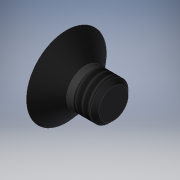
# Autodesk Inventor part: FBb4-5
Saved by Autodesk Inventor 2019 (Build 230136000, 136)
## iProperties
Created: 2024-03-12
Part Number: FBb4-5
Material: Generic
Catalog Web Link: www.cadenas.de
Description: FBb-Cross Recessed Countersunk Head Screw
Vendor: MISUMI
Document SubType Name: Modeling
Designer: psAdmin
Manufacturer: MISUMI
Mass: 0.0947838 g
Surface Area: 1.75917 cm^2
Volume: 0.0947838 cm^3
Density: 1 g/cm^3
Appearance: PSOLRGB-175-175-175
Category: PARTsolutions
Company: MISUMI
Title: FBb4-5
Author: Cadenas PARTsolutions
Comments: Cross Recessed Countersunk Head Screw
PSOL_IDENT_0: {$CADENAS_DATA/23d-libs/misumi/metric/28_keys_magnets/fb_b.prj},152 {VTYP=3D},{NB=FBb4-5},{LINA=FBb4
PSOL_IDENT_1: -5},{NN=FBb},{DATE=06.04.2023 02:31:49},{GEOMDATE=29.03.2023 02:05:00},{VERSION=},{LINEID=160},{WBVA
PSOL_IDENT_2: R=L},{WBNUMERIC=L}  {NB=FBb4-5},{LINA=FBb4-5},{KT=DUMMY},{PN=FBb4-5},{MAT=4137 Steel},{HARD=32~38HRC
PSOL_IDENT_3: },{M=4.0},{L=5},{LL=Full Thread},{L1=14},{TYPE=FBb},{L0=[3:50/1]},{NDM=4},{KDM=3.139931},{MP=4x0.7},
PSOL_IDENT_4: {P=0.700},{A=8.500},{E=2.00},{B=2.50},{E0=3}
NB: FBb4-5
NN: FBb
NT: Cross Recessed Countersunk Head Screw
NBSYN: $PN.
LINA: FBb4-5
CATALOG: Misumi
PN: FBb4-5
MAT: 4137 Steel
HARD: 32~38HRC
M: 4
L: 5
LL: Full Thread
MP: 4x0.7
P: 0.7
A: 8.5
B: 2.5
SUPPLIER: MISUMI
ARTICLENO: FBb4-5
BOMINFO: FBb4-5
CREATOR: CADENAS GmbH
Autodesk Inventor part; units mm, degrees
sketch "Sketch_1" plane through (0, 0, 0) normal (0, 0, 1) x (1, 0, 0)
  line L0 (5, 0) -> (0, 0)
  line L1 (0, 0) -> (0, 4.25)
  line L2 (0, 4.25) -> (2, 2)
  line L3 (2, 2) -> (4.5705, 2)
  line L4 (4.5705, 2) -> (5, 1.5705)
  line L5 (5, 1.5705) -> (5, 0)
  line L6 (5, 0) -> (0, 0)
  constraints: 14 end point
revolve "Revolution1" add sketch "Sketch_1" angle 360 about axis through (5, 0, 0) along (1, 0, 0)
thread "Thread1" size "M4x0.7" class "6g" standard "ISO Metric profile" length 1.8266
sketch "_____1" plane through (0, 0, 0) normal (1, 0, 0) x (0, 0, -1)
  line L0 (-1.75, 0.4667) -> (-1.75, -0.4667)
  line L1 (-1.75, -0.4667) -> (-0.9333, -0.4667)
  arc A0 (-0.4667, -0.9333) -> (-0.9333, -0.4667) centre (-0.9333, -0.9333) ccw
  line L2 (-0.4667, -0.9333) -> (-0.4667, -1.75)
  line L3 (-0.4667, -1.75) -> (0.4667, -1.75)
  line L4 (0.4667, -1.75) -> (0.4667, -0.9333)
  arc A1 (0.9333, -0.4667) -> (0.4667, -0.9333) centre (0.9333, -0.9333) ccw
  line L5 (0.9333, -0.4667) -> (1.75, -0.4667)
  line L6 (1.75, -0.4667) -> (1.75, 0.4667)
  line L7 (1.75, 0.4667) -> (0.9333, 0.4667)
  arc A2 (0.4667, 0.9333) -> (0.9333, 0.4667) centre (0.9333, 0.9333) ccw
  line L8 (0.4667, 0.9333) -> (0.4667, 1.75)
  line L9 (0.4667, 1.75) -> (-0.4667, 1.75)
  line L10 (-0.4667, 1.75) -> (-0.4667, 0.9333)
  arc A3 (-0.9333, 0.4667) -> (-0.4667, 0.9333) centre (-0.9333, 0.9333) ccw
  line L11 (-0.9333, 0.4667) -> (-1.75, 0.4667)
  constraints: 24 end point, 8 point on circle, 4 centre point
extrude "Extrusion1" cut sketch "_____1" along normal blind 1
ref_plane "screw_XY" through (2, 0, 0) normal (1, 0, 0) x (0, 0, -1)
ref_plane "screw_YZ" through (2, 0, 0) normal (0, 0, -1) x (0, 1, 0)
ref_plane "screw_ZX" through (2, 0, 0) normal (0, 1, 0) x (1, 0, 0)
body "Solid1"
